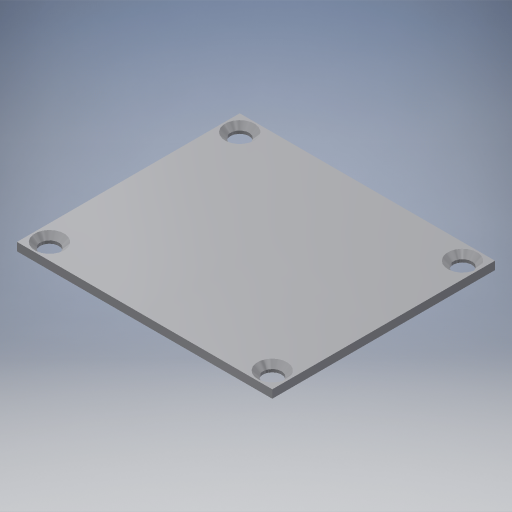
# Autodesk Inventor part: Mixer IQ Box ND20
Saved by Autodesk Inventor 2024 (Build 280153000, 153)
## iProperties
Created: 2009-10-07
Part Number: Mixer IQ Box ND20
Material: Aluminum-6061
Document SubType Name: Modeling
Designer: M. Brock
Mass: 13.5075 g
Surface Area: 35.786 cm^2
Volume: 4.98432 cm^3
Density: 2.71 g/cm^3
Appearance: Aluminum - Flat
Author: M. Brock
Autodesk Inventor part; units mm, degrees
ref_plane "YZ Plane" through (0, 0, 0) normal (1, 0, 0) x (0, 1, 0)
ref_plane "XZ Plane" through (0, 0, 0) normal (0, 1, 0) x (-1, 0, 0)
ref_plane "XY Plane" through (0, 0, 0) normal (0, 0, 1) x (1, 0, 0)
sketch "Sketch1" plane through (0, 0, 0) normal (0, 0, 1) x (1, 0, 0)
  line L0 (0, 0) -> (31.4, 0)
  line L1 (31.4, 0) -> (31.4, 27.4)
  line L2 (31.4, 27.4) -> (0, 27.4)
  line L3 (0, 27.4) -> (0, 0)
  dimension "d0" = 31.4
  dimension "d1" = 27.4
  constraints: 8 end point, 2 parallel, 1 horizontal, 1 perpendicular
  measures "d0" distance between parallel lines of L3 L1
  measures "d1" distance between parallel lines of L2 L0
extrude "Extrusion1" add sketch "Sketch1" along normal blind 1
sketch "Sketch17" plane through (0, 0, 1) normal (0, 0, 1) x (1, 0, 0)
  line L0 (2, 25.4) -> (29.4, 25.4) construction
  line L1 (29.4, 25.4) -> (29.4, 2) construction
  line L2 (29.4, 2) -> (2, 2) construction
  line L3 (2, 2) -> (2, 25.4) construction
  line L4 (0, 0) -> (0, 27.4) construction
  line L5 (0, 27.4) -> (31.4, 27.4) construction
  dimension "d169" = 27.4
  dimension "d170" = 23.4
  dimension "d171" = 2
  dimension "d172" = 2
  constraints: 8 end point, 4 coincident, 2 parallel, 1 horizontal, 1 perpendicular
  measures "d169" distance of L1.end L2.end
  measures "d170" distance of L0.end L1.end
  measures "d171" distance between parallel lines of L4 L3
  measures "d172" distance between parallel lines of L5 L0
hole "Hole16" at (2, 25.4, 1) at (29.4, 25.4, 1) at (29.4, 2, 1) at (2, 2, 1) direction (0, 0, -1) diameter 2.3 end through all countersink diameter 3.6 countersink angle 90
body "Solid1"
